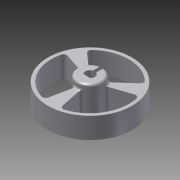
# Autodesk Inventor part: Roue
Saved by Autodesk Inventor 2014 SP2 (Build 180246200, 246)
## iProperties
Created: 2015-03-17
Part Number: Roue
Material: Plastique ABS
Document SubType Name: Modeling
Designer: sd
Density: 1.06 g/cm^3
Appearance: Lisse - Blanc
Mass: 1.44291 g
Surface Area: 18.7913 cm^2
Volume: 1.36124 cm^3
Author: sd
Autodesk Inventor part; units mm, degrees
ref_plane "YZ Plane" through (0, 0, 0) normal (1, 0, 0) x (0, 1, 0)
ref_plane "XZ Plane" through (0, 0, 0) normal (0, 1, 0) x (-1, 0, 0)
ref_plane "XY Plane" through (0, 0, 0) normal (0, 0, 1) x (1, 0, 0)
sketch "Esquisse1" plane through (0, 0, 0) normal (0, 0, 1) x (1, 0, 0)
  circle A0 centre (0, 0) radius 13
  dimension "d0" = 26
  constraints: 1 centre point, 1 coincident
  measures "d0" diameter of A0
extrude "Extrusion1" add sketch "Esquisse1" along normal blind 6.5
sketch "Esquisse2" plane through (0, 0, 6.5) normal (0, 0, 1) x (1, 0, 0)
  circle A0 centre (0, 0) radius 13 projected
  line L0 (0, 0) -> (-9, 8)
  line L1 (0, 0) -> (9, 8)
  arc A1 (9, 8) -> (-9, 8) centre (0, -0.125) ccw
  arc A2 (2.9268, 2.6016) -> (-2.9268, 2.6016) centre (0, -0.125) ccw
  dimension "d3" = 8
  dimension "d4" = 8
  dimension "d5" = 9
  dimension "d6" = 9
  dimension "d7" = 1
  dimension "d8" = 4
  constraints: 4 end point, 4 point on circle, 2 centre point, 2 point on line, 1 concentric
  measures "d3" vertical distance of L0.start L0.end
  measures "d4" vertical distance of L0.start L1.end
  measures "d5" horizontal distance of L0.start L1.end
  measures "d6" horizontal distance of L0.start L0.end
  measures "d8" distance of A1.centre A2.end
extrude "Extrusion2" cut sketch "Esquisse2" against normal through all contours L0 A1 L1 A2
fillet "Congé1" radius 1 4 edges at (-9, 8, 3.25) (9, 8, 3.25) (-2.9268, 2.6016, 3.25) (2.9268, 2.6016, 3.25)
pattern_circular "Réseau circulaire1" count 3 over 360 about axis through (0, 0, 0) along (0, 0, 1) of "Extrusion2"
fillet "Congé2" radius 1 8 edges at (-11.4282, 3.7942, 3.25) (-3.7164, 1.2339, 3.25) (11.4282, 3.7942, 3.25) (0.7896, -3.8354, 3.25) (-0.7896, -3.8354, 3.25) (2.4282, -11.7942, 3.25) (-2.4282, -11.7942, 3.25) (3.7164, 1.2339, 3.25)
sketch "Esquisse3" plane through (0, 0, 6.5) normal (0, 0, 1) x (1, 0, 0)
  circle A0 centre (0, 0) radius 13 projected
  circle A1 centre (0, 0) radius 3.9413
  constraints: 1 centre point, 1 coincident
extrude "Extrusion3" add sketch "Esquisse3" along normal blind 2 contours A1
fillet "Congé3" radius 0.7 1 edges at (-3.9413, 0, 8.5)
fillet "Congé4" radius 0.6 3 edges at (-3.4133, 1.9707, 6.5) (3.4133, 1.9707, 6.5) (0, -3.9413, 6.5)
sketch "Esquisse4" plane through (0, 0, 8.5) normal (0, 0, 1) x (1, 0, 0)
  circle A0 centre (0, 0) radius 3.2413 projected
  circle A1 centre (0, 0) radius 1.5
  line L0 (-0.5, 1.4142) -> (-0.5, 4.5)
  line L1 (-0.5, 4.5) -> (0.5, 4.5)
  line L2 (0.5, 4.5) -> (0.5, 1.4142)
  line L3 (-1.118, -1) -> (1.118, -1)
  dimension "d20" = 3
  dimension "d21" = 1
  dimension "d22" = 0.5
  dimension "d23" = 4.5
  dimension "d24" = 2.5
  constraints: 8 end point, 4 point on circle, 2 perpendicular, 1 centre point, 1 coincident, 1 parallel, 1 vertical
  measures "d20" diameter of A1
  measures "d21" distance between parallel lines of L2 L0
  measures "d22" distance from line of A0.centre L0
  measures "d23" distance from line of A0.centre L1
extrude "Extrusion4" cut sketch "Esquisse4" against normal through all contours L2 A1 L0 A0 | A0 L0 L1 L2 | A1 L3 picked at (-0.0558, 2.0726) picked at (0.0565, -0.1699)
equation "\"d22\" = 0.5 * d21"
